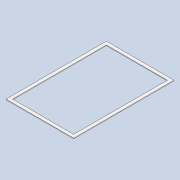
# Autodesk Inventor part: Marco molde
Saved by Autodesk Inventor 2021 (Build 250183000, 183)
## iProperties
Created: 2021-04-17
Part Number: Marco molde
Material: Genérico
Document SubType Name: Modeling
Designer: Admin
Density: 1 g/cm^3
Appearance: Blanco
Author: Admin
Autodesk Inventor part; units mm, degrees
ref_plane "YZ Plane" through (0, 0, 0) normal (1, 0, 0) x (0, 1, 0)
ref_plane "XZ Plane" through (0, 0, 0) normal (0, 1, 0) x (-1, 0, 0)
ref_plane "XY Plane" through (0, 0, 0) normal (0, 0, 1) x (1, 0, 0)
sketch "Boceto1" plane through (0, 0, 0) normal (0, 1, 0) x (-1, 0, 0)
  line L0 (0, 0) -> (280, 0)
  line L1 (280, 0) -> (280, -430)
  line L2 (280, -430) -> (0, -430)
  line L3 (0, -430) -> (0, 0)
  line L4 (0, 15) -> (295, 15)
  line L5 (295, 15) -> (295, -445)
  line L6 (295, -445) -> (-15, -445)
  line L7 (-15, -445) -> (-15, 15)
  line L8 (-15, 15) -> (0, 15)
  dimension "d0" = 280
  dimension "d1" = 430
  dimension "d2" = 15
  dimension "d3" = 295
  dimension "d4" = 460
  dimension "d5" = 310
  constraints: 18 end point, 5 perpendicular, 2 horizontal, 2 parallel, 1 point on line
  measures "d0" distance of L1.end L2.end
  measures "d1" distance of L0.end L1.end
  measures "d2" distance of L0.start L4.start
  measures "d3" distance of L4.start L4.end
  measures "d4" distance of L4.end L5.end
  measures "d5" distance of L5.end L6.end
extrude "Extrusión1" add sketch "Boceto1" along normal blind 3
